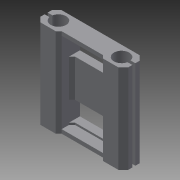
# Autodesk Inventor part: ChimeraXCarriageFanBottom
Saved by Autodesk Inventor 2015 SP1 (Build 190203100, 203)
## iProperties
Created: 2014-12-18
Part Number: ChimeraXCarriageFanBottom
Material: Generic
Document SubType Name: Modeling
Designer: Jack
Density: 1 g/cm^3
Appearance: Default
Author: Jack
Autodesk Inventor part; units mm, degrees
ref_plane "YZ Plane" through (0, 0, 0) normal (1, 0, 0) x (0, 1, 0)
ref_plane "XZ Plane" through (0, 0, 0) normal (0, 1, 0) x (-1, 0, 0)
ref_plane "XY Plane" through (0, 0, 0) normal (0, 0, 1) x (1, 0, 0)
sketch "Sketch1" plane through (0, 0, 0) normal (0, 0, 1) x (1, 0, 0)
  arc A0 (-7.6035, -1.5) -> (-7.6035, 1.5) centre (0, 0) ccw
  arc A1 (71.6035, 1.5) -> (71.6035, -1.5) centre (64, 0) ccw
  line L0 (-12.5, 10.75) -> (76.5, 10.75)
  line L1 (76.5, -10.75) -> (-12.5, -10.75)
  line L2 (-12.5, 1.5) -> (-7.6035, 1.5)
  line L3 (-12.5, -1.5) -> (-7.6035, -1.5)
  line L4 (-12.5, -10.75) -> (-12.5, -1.5)
  line L5 (-12.5, 1.5) -> (-12.5, 10.75)
  line L6 (76.5, 1.5) -> (71.6035, 1.5)
  line L7 (76.5, -1.5) -> (71.6035, -1.5)
  line L8 (76.5, 10.75) -> (76.5, 1.5)
  line L9 (76.5, -1.5) -> (76.5, -10.75)
  dimension "d0" = 15.5
  dimension "d1" = 15.5
  dimension "d2" = 64
  dimension "d3" = 10.75
  dimension "d4" = 10.75
  dimension "d5" = 1.5
  dimension "d6" = 3
  dimension "d7" = 12.5
  dimension "d8" = 12.5
  constraints: 20 end point, 6 perpendicular, 4 point on circle, 3 horizontal, 3 horizontal alignment, 2 centre point, 2 coincident, 2 vertical, 2 vertical alignment, 1 parallel
  measures "d0" diameter of A0
  measures "d1" diameter of A1
  measures "d2" distance of point (0, 0) A1.centre
  measures "d3" distance from line of point (0, 0) L1
  measures "d4" distance from line of L0 point (0, 0)
  measures "d5" distance from line of A1.centre L7
  measures "d6" distance between parallel lines of L6 L7
  measures "d7" distance from line of point (0, 0) L5
  measures "d8" distance from line of L8 A1.centre
extrude "Extrusion1" add sketch "Sketch1" along normal blind 90
chamfer "Chamfer1" distance 5 angle 45 4 edges at (-12.5, 10.75, 45) (-12.5, -10.75, 45) (76.5, 10.75, 45) (76.5, -10.75, 45)
sketch "Sketch2" plane through (0, 0, 90) normal (0, 0, 1) x (1, 0, 0)
  arc A0 (71.6035, 1.5) -> (71.6035, -1.5) centre (64, 0) ccw projected
  line L0 (71.5, 10.75) -> (-7.5, 10.75) projected
  arc A1 (-7.6035, -1.5) -> (-7.6035, 1.5) centre (0, 0) ccw projected
  line L1 (-7.5, -10.75) -> (71.5, -10.75) projected
  line L2 (11, -10.75) -> (11, 2.75)
  line L3 (11, 2.75) -> (53, 2.75)
  line L4 (53, 2.75) -> (53, -10.75)
  dimension "d14" = 8
  dimension "d15" = 11
  dimension "d16" = 11
  constraints: 6 end point, 2 perpendicular, 2 point on line, 1 vertical
  measures "d14" distance between parallel lines of L0 L3
  measures "d15" distance from line of A0.centre L4
  measures "d16" distance from line of A1.centre L2
extrude "Extrusion2" cut sketch "Sketch2" against normal up to next
chamfer "Chamfer2" distance 3 angle 45 2 edges at (11, 2.75, 45) (53, 2.75, 45)
sketch "Sketch5" plane through (0, 0, 90) normal (0, 0, 1) x (1, 0, 0)
  line L0 (11, -10.75) -> (11, -0.25) projected
  line L1 (14, 2.75) -> (11, -0.25) projected
  line L2 (14, 2.75) -> (50, 2.75) projected
  line L3 (53, -0.25) -> (50, 2.75) projected
  line L4 (53, -0.25) -> (53, -10.75) projected
  line L5 (53, -10.75) -> (71.5, -10.75) projected
  line L6 (11, -7.75) -> (53, -7.75)
  dimension "d28" = 3
  constraints: 2 end point, 2 point on line, 1 perpendicular
  measures "d28" distance between parallel lines of L5 L6
extrude "Extrusion5" add sketch "Sketch5" against normal blind 4
sketch "Sketch6" plane through (0, 0, 0) normal (0, 0, -1) x (-1, 0, 0)
  line L0 (-11, -0.25) -> (-11, -10.75) projected
  line L1 (-53, -10.75) -> (-53, -0.25) projected
  line L2 (-50, 2.75) -> (-53, -0.25) projected
  line L3 (-50, 2.75) -> (-14, 2.75) projected
  line L4 (-11, -0.25) -> (-14, 2.75) projected
  line L5 (-53, -7.75) -> (-11, -7.75) projected
extrude "Extrusion6" add sketch "Sketch6" against normal blind 4
chamfer "Chamfer3" distance 3 angle 45 2 edges at (11, -10.75, 45) (53, -10.75, 45)
sketch "Sketch9" plane through (14, 2.75, 86) normal (0, -1, 0) x (1, 0, 0)
  line L0 (0, -82) -> (36, -82) projected
  line L1 (36, 0) -> (36, -82) projected
  line L2 (36, 0) -> (0, 0) projected
  line L3 (36, -82) -> (39, -82) projected
  line L4 (39, -82) -> (39, 0) projected
  line L5 (39, 0) -> (36, 0) projected
  line L6 (36, 0) -> (36, -82) projected
  line L7 (-3, -82) -> (0, -82) projected
  line L8 (0, -82) -> (0, 0) projected
  line L9 (0, 0) -> (-3, 0) projected
  line L10 (-3, 0) -> (-3, -82) projected
  line L11 (39, 0) -> (39, -82) projected
  line L12 (39, -82) -> (39, 0) projected
  line L13 (39, -2) -> (-3, -2)
  line L14 (39, -22) -> (-3, -22)
  line L15 (-3, 0) -> (-3, -82) projected
  line L16 (-3, -60) -> (39, -60)
  line L17 (39, -80) -> (-3, -80)
  point P0 (-14, -86)
  dimension "d47" = 2
  dimension "d48" = 2
  dimension "d49" = 20
  dimension "d50" = 20
  constraints: 8 end point, 8 point on line, 3 perpendicular, 1 parallel
  measures "d47" distance between parallel lines of L2 L13
  measures "d48" distance between parallel lines of L0 L17
  measures "d49" distance between parallel lines of L17 L16
  measures "d50" distance between parallel lines of L13 L14
extrude "Extrusion9" cut sketch "Sketch9" along normal blind 3 and the other way blind 8 contours L17 L10 L16 L8 | L8 L16 L1 L17 | L1 L16 L4 L17 | L14 L10 L13 L8 | L8 L13 L1 L14 | L1 L13 L4 L14
sketch "Sketch7" plane through (0, 0, 12) normal (0, 0, 1) x (1, 0, 0)
  circle A0 centre (14.5, -0.75) radius 1.5
  circle A1 centre (49.5, -0.75) radius 1.5
  line L0 (14, 2.75) -> (50, 2.75) projected
  line L1 (53, -0.25) -> (53, -7.75) projected
  line L2 (50, 2.75) -> (53, -0.25) projected
  line L3 (11, -0.25) -> (14, 2.75) projected
  arc A2 (46.6716, -0.75) -> (49.5, -3.5784) centre (49.5, -0.75) ccw
  line L4 (49.5, -3.5784) -> (53, -3.5784)
  arc A3 (14.5, -3.5784) -> (17.3284, -0.75) centre (14.5, -0.75) ccw
  line L5 (14.5, -3.5784) -> (11, -3.5784)
  line L6 (11, -7.75) -> (11, -0.25) projected
  line L7 (17.3284, -0.75) -> (17.3284, 2.75)
  line L8 (46.6716, -0.75) -> (46.6716, 2.75)
  point P0 (0, 0)
  dimension "d37" = 3
  dimension "d38" = 3
  dimension "d39" = 3.5
  dimension "d40" = 35
  dimension "d41" = 3.5
  constraints: 8 end point, 6 tangent, 4 centre point, 4 point on circle, 4 point on line, 2 coincident, 2 horizontal, 2 perpendicular, 1 horizontal alignment
  measures "d37" diameter of A0
  measures "d38" diameter of A1
  measures "d39" distance from line of L0 A1.centre
  measures "d40" distance of A0.centre A1.centre
  measures "d41" distance from line of L1 A1.centre
sketch "Sketch8" plane through (0, 0, 78) normal (0, 0, -1) x (-1, 0, 0)
  circle A0 centre (-49.5, -0.75) radius 1.5 projected
  line L0 (-46.6716, 2.75) -> (-46.6716, -0.75) projected
  arc A1 (-49.5, -3.5784) -> (-46.6716, -0.75) centre (-49.5, -0.75) ccw projected
  line L1 (-49.5, -3.5784) -> (-53, -3.5784) projected
  line L2 (-53, -0.25) -> (-53, -3.5784) projected
  line L3 (-50, 2.75) -> (-53, -0.25) projected
  line L4 (-46.6716, 2.75) -> (-50, 2.75) projected
  circle A2 centre (-14.5, -0.75) radius 1.5 projected
  line L5 (-11, -0.25) -> (-14, 2.75) projected
  line L6 (-11, -3.5784) -> (-11, -0.25) projected
  line L7 (-11, -3.5784) -> (-14.5, -3.5784) projected
  arc A3 (-17.3284, -0.75) -> (-14.5, -3.5784) centre (-14.5, -0.75) ccw projected
  line L8 (-17.3284, -0.75) -> (-17.3284, 2.75) projected
  line L9 (-14, 2.75) -> (-17.3284, 2.75) projected
  point P0 (0, 0)
body "Solid1"
